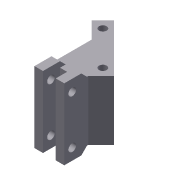
# Autodesk Inventor part: Knee - Back
Saved by Autodesk Inventor 2011 (Build 150239000, 239)
## iProperties
Created: 2010-11-21
Part Number: Knee - Back
Document SubType Name: Modeling
Designer: Milton
Density: 2.71 g/cm^3
Mass: 14.6327 g
Surface Area: 30.6725 cm^2
Volume: 5.39951 cm^3
Material: Aluminum-6061
Author: Milton
Autodesk Inventor part; units mm, degrees
ref_plane "YZ Plane" through (0, 0, 0) normal (1, 0, 0) x (0, 1, 0)
ref_plane "XZ Plane" through (0, 0, 0) normal (0, 1, 0) x (-1, 0, 0)
ref_plane "XY Plane" through (0, 0, 0) normal (0, 0, 1) x (1, 0, 0)
sketch "Sketch1" plane through (0, 0, 0) normal (0, 0, 1) x (1, 0, 0)
  line L0 (13.7683, -3.4584) -> (10.7683, -3.4584)
  line L1 (13.7683, -3.4584) -> (13.7683, 2.5416)
  circle A0 centre (9.3262, 22.064) radius 1.35
  circle A1 centre (21.3453, 10.0416) radius 1.35
  line L2 (10.7683, -3.4584) -> (13.7683, -3.4584)
  line L3 (9.4532, 26.0885) -> (40.2875, 26.0885) construction
  line L4 (13.7683, 2.5416) -> (18.2683, 2.5416)
  line L5 (10.7683, 16.6612) -> (10.7683, -3.4584)
  line L6 (26.507, 8.8387) -> (-1.0663, 36.4198) projected
  arc A2 (26.507, 8.8387) -> (30.7497, 8.8382) centre (28.6286, 10.9598) ccw projected
  line L7 (28.2745, 6.3636) -> (30.7497, 8.8382) projected
  line L8 (28.2745, 6.3636) -> (20.4257, 7.0011) projected
  line L9 (20.4257, 7.0011) -> (-6.8649, 34.2993) projected
  line L10 (-6.8649, 34.2993) -> (-7.5002, 42.1482) projected
  line L11 (-7.5002, 42.1482) -> (10.4629, 60.1062) projected
  line L12 (10.4629, 60.1062) -> (18.3117, 59.4687) projected
  line L13 (18.3117, 59.4687) -> (45.6022, 32.1706) projected
  line L14 (45.6022, 32.1706) -> (46.2375, 24.3216) projected
  line L15 (43.7623, 21.8471) -> (46.2375, 24.3216) projected
  arc A3 (43.7623, 21.8471) -> (43.7628, 26.0897) centre (41.6412, 23.9687) ccw projected
  line L16 (16.1895, 53.6708) -> (43.7628, 26.0897) projected
  arc A4 (16.1895, 53.6708) -> (11.9469, 53.6714) centre (14.0679, 51.5497) ccw projected
  line L17 (-1.0657, 40.6624) -> (11.9469, 53.6714) projected
  arc A5 (-1.0657, 40.6624) -> (-1.0663, 36.4198) centre (1.0553, 38.5408) ccw projected
  line L18 (26.507, 8.8387) -> (-1.0663, 36.4198) projected
  circle A6 centre (18.5232, 55.2968) radius 1.35 projected
  circle A7 centre (-2.693, 34.0865) radius 1.35 projected
  circle A8 centre (9.4722, 55.1566) radius 1.35 projected
  circle A9 centre (30.5424, 43.2743) radius 1.35 projected
  circle A10 centre (42.5615, 31.2518) radius 1.35 projected
  circle A11 centre (-2.5503, 43.1375) radius 1.35 projected
  circle A12 centre (9.3262, 22.064) radius 1.35 projected
  circle A13 centre (21.3453, 10.0416) radius 1.35 projected
  line L19 (4.8715, 22.5596) -> (8.8318, 26.5189)
  line L20 (8.8318, 26.5189) -> (25.8, 9.546)
  line L21 (4.8715, 22.5596) -> (10.7683, 16.6612)
  line L22 (18.2683, -2.9731) -> (18.2683, 2.1519) projected
  line L23 (18.2683, 2.5416) -> (18.2683, -3.4584)
  line L24 (18.2683, -3.4584) -> (21.2683, -3.4584)
  line L25 (21.2683, -3.4584) -> (21.2683, 5.0155)
  line L26 (25.8, 9.546) -> (21.2683, 5.0155)
  point P0 (0, 0)
  dimension "d9" = 2.7
  dimension "d10" = 2.7
  dimension "d12" = 3
  dimension "d28" = 6
  dimension "d35" = 3.5
  dimension "d36" = 24
  dimension "d38" = 3
  dimension "d63" = 4.5
  constraints: 26 end point, 4 perpendicular, 4 point on line, 2 centre point, 2 concentric, 2 horizontal, 2 vertical, 1 collinear, 1 parallel, 1 point on circle
  measures "d9" diameter of A0
  measures "d10" diameter of A1
  measures "d12" distance of L0.start L0.end
  measures "d28" distance between parallel lines of L0 L4
  measures "d35" distance from line of A12.centre L19
  measures "d36" distance of L19.end L20.end
  measures "d38" distance of L23.end L24.end
  measures "d63" distance of L1.end L4.end
extrude "Extrusion1" add sketch "Sketch1" along normal blind 25 contours L0 L5 L9 L8 L26 L25 L24 L23 L22 L4 L1 | L9 L19 L6 L26 L8
sketch "Sketch3" plane through (10.7683, -3.4584, 0) normal (-1, 0, 0) x (0, 0, 1)
  circle A0 centre (2, 2.8104) radius 1.35 projected
  circle A1 centre (19, 2.8104) radius 1.35 projected
  line L0 (25, 0) -> (25, 20.1196) projected
  line L1 (0, 20.1196) -> (0, 0) projected
  circle A2 centre (4, 2.8104) radius 1.35
  circle A3 centre (21, 2.8104) radius 1.35
  dimension "d48" = 2.7
  dimension "d49" = 2.7
  dimension "d50" = 4
  dimension "d51" = 4
  constraints: 2 centre point
  measures "d48" diameter of A2
  measures "d49" diameter of A3
  measures "d50" distance from line of L1 A2.centre
  measures "d51" distance from line of L0 A3.centre
extrude "Extrusion3" cut sketch "Sketch3" against normal through all contours A0 A2 | A0 A2 | A1 A3 | A1 A3 picked at (3.1032, 2.701) picked at (4.6704, 2.7032) picked at (20.1032, 2.9198) picked at (21.6704, 2.9176)
sketch "Sketch5" plane through (10.7683, -3.4584, 0) normal (-1, 0, 0) x (0, 0, 1)
  line L0 (0, 0) -> (25, 0) projected
  line L1 (0, 0) -> (0, 8.4739) projected
  line L2 (0, 6) -> (2, 6)
  line L3 (2, 6) -> (2, 32)
  line L4 (2, 32) -> (0, 32)
  line L5 (0, 32) -> (0, 6)
  line L6 (25, 8.4739) -> (25, 0) projected
  line L7 (25, 6) -> (23, 6)
  line L8 (23, 6) -> (23, 32)
  line L9 (23, 32) -> (25, 32)
  line L10 (25, 32) -> (25, 6)
  point P0 (0, 3.4584)
  dimension "d52" = 2
  dimension "d53" = 26
  dimension "d54" = 6
  dimension "d55" = 2
  dimension "d56" = 26
  dimension "d57" = 6
  constraints: 16 end point, 4 parallel, 2 horizontal, 2 perpendicular, 2 point on line
  measures "d52" distance of L4.end L3.end
  measures "d53" distance of L3.end L2.end
  measures "d54" distance between parallel lines of L0 L2
  measures "d55" distance of L8.end L9.end
  measures "d56" distance of L7.end L8.end
  measures "d57" distance between parallel lines of L0 L7
extrude "Extrusion4" cut sketch "Sketch5" along normal through all both and the other way through all
chamfer "Chamfer1" distance 2 angle 45 4 edges at (12.2683, 2.5416, 23) (19.7683, 2.5416, 23) (19.7683, 2.5416, 2) (12.2683, 2.5416, 2)
body "Solid1"
